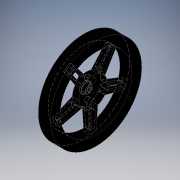
# Autodesk Inventor part: wheel
Saved by Autodesk Inventor 2016 (Build 200138000, 138)
## iProperties
Created: 2016-01-12
Part Number: wheel
Material: Generic
Document SubType Name: Modeling
Designer: jferner
Density: 1 g/cm^3
Appearance: Default
Author: jferner
Autodesk Inventor part; units mm, degrees
ref_plane "YZ Plane" through (0, 0, 0) normal (1, 0, 0) x (0, 1, 0)
sketch "Sketch1" plane through (0, 0, 0) normal (1, 0, 0) x (0, 1, 0)
  circle A0 centre (0, 0) radius 30
  circle A1 centre (0, 0) radius 23.65
  dimension "wheelDiameter" = 60
  dimension "wheelInnerDiameter" = 47.3
  constraints: 2 centre point, 2 coincident
  measures "wheelDiameter" diameter of A0
  measures "wheelInnerDiameter" diameter of A1
extrude "Extrusion1" add sketch "Sketch1" along normal mid plane 8
sketch "Sketch2" plane through (0, 0, 0) normal (1, 0, 0) x (0, 1, 0)
  circle A0 centre (0, 0) radius 9.4
  dimension "hubOuterDiameter" = 18.8
  constraints: 1 centre point, 1 coincident
  measures "hubOuterDiameter" diameter of A0
extrude "Extrusion2" add sketch "Sketch2" along normal mid plane 4.3
sketch "Sketch3" plane through (-2.15, 0, 0) normal (-1, 0, 0) x (0, 0, 1)
  circle A0 centre (0, 0) radius 1.22
  dimension "d7" = 2.44
  constraints: 1 centre point, 1 coincident
  measures "d7" diameter of A0
extrude "Extrusion3" cut sketch "Sketch3" against normal through all
sketch "Sketch4" plane through (-2.15, 0, 0) normal (-1, 0, 0) x (0, 0, 1)
  circle A0 centre (-6.3, 0) radius 1.6
  point P0 (0, 0)
  dimension "d10" = 3.2
  dimension "d11" = 6.3
  constraints: 1 centre point
  measures "d10" diameter of A0
  measures "d11" distance of point (0, 0) A0.centre
extrude "Extrusion4" cut sketch "Sketch4" against normal through all
pattern_circular "Circular Pattern1" count 2 over 360 about axis through (-2.15, 0, 0) along (1, 0, 0) of "Extrusion4"
sketch "Sketch5" plane through (-2.15, 0, 0) normal (-1, 0, 0) x (0, 0, 1)
  circle A0 centre (0, 0) radius 2.3
  circle A1 centre (0, 0) radius 1.22 projected
  circle A2 centre (0, 0) radius 3.5
  dimension "servoShaftDiameter" = 4.6
  dimension "d18" = 7
  constraints: 2 centre point, 2 coincident
  measures "servoShaftDiameter" diameter of A0
  measures "d18" diameter of A2
extrude "Extrusion5" add sketch "Sketch5" along normal blind 1.14 contours A2
sketch "Sketch7" plane through (-3.29, 0, 0) normal (-1, 0, 0) x (0, 0, 1)
  circle A0 centre (0, 0) radius 2.3
  dimension "d23" = 4.6
  constraints: 1 centre point, 1 coincident
  measures "d23" diameter of A0
extrude "Extrusion6" cut sketch "Sketch7" against normal blind 2.5
ref_plane "Work Plane2" through (0, 0, -9.4) normal (0, 0, 1) x (1, 0, 0)
sketch "Sketch9" plane through (0, 0, -9.4) normal (0, 0, 1) x (1, 0, 0)
  line L0 (2.15, 2.9) -> (-2.15, 2.9)
  line L1 (-2.15, 2.9) -> (-2.15, -2.9)
  line L2 (-2.15, -2.9) -> (2.15, -2.9)
  line L3 (2.15, -2.9) -> (2.15, 2.9)
  point P0 (0, 0)
  dimension "d24" = 2.15
  dimension "d25" = 4.3
  dimension "d26" = 5.8
  dimension "d27" = 2.9
  constraints: 8 end point, 2 parallel, 1 horizontal, 1 perpendicular
  measures "d24" distance from line of L1 point (0, 0)
  measures "d25" distance between parallel lines of L1 L3
  measures "d26" distance between parallel lines of L2 L0
  measures "d27" distance from line of L0 point (0, 0)
ref_plane "Work Plane3" through (0, 0, -23.65) normal (0, 0, 1) x (1, 0, 0)
sketch "Sketch10" plane through (0, 0, -23.65) normal (0, 0, 1) x (1, 0, 0)
  line L0 (-1.5, 2.5) -> (1.5, 2.5)
  line L1 (1.5, 2.5) -> (1.5, -2.5)
  line L2 (1.5, -2.5) -> (-1.5, -2.5)
  line L3 (-1.5, -2.5) -> (-1.5, 2.5)
  line L4 (0, 0) -> (2.563972, 0)
  line L5 (0, 0) -> (0, 2.208122)
  dimension "d28" = 3
  dimension "d29" = 5
  constraints: 12 end point, 2 horizontal, 2 parallel, 1 perpendicular, 1 vertical, 2 other
  measures "d28" distance between parallel lines of L1 L3
  measures "d29" distance of L0.end L1.end
sketch "Sketch10 outline for Loft1" plane through (0, 0, -23.65) normal (0, 0, 1) x (1, 0, 0)
  line L0 (-1.5, 2.5) -> (1.5, 2.5)
  line L1 (1.5, 2.5) -> (1.5, -2.5)
  line L2 (1.5, -2.5) -> (-1.5, -2.5)
  line L3 (-1.5, -2.5) -> (-1.5, 2.5)
sketch "Sketch9 outline for Loft1" plane through (0, 0, -9.4) normal (0, 0, 1) x (1, 0, 0)
  line L0 (2.15, -2.9) -> (2.15, 2.9)
  line L1 (-2.15, -2.9) -> (2.15, -2.9)
  line L2 (-2.15, 2.9) -> (-2.15, -2.9)
  line L3 (2.15, 2.9) -> (-2.15, 2.9)
loft "Loft1" add profiles "Sketch10 outline for Loft1", "Sketch9 outline for Loft1"
sketch "Sketch11" plane through (-2.15, 0, 0) normal (-1, 0, 0) x (0, 0, 1)
  line L0 (-23.517097, 2.503731) -> (-9.4, 2.9)
  line L1 (-9.4, 2.9) -> (-8.937253, 2.912989)
  circle A0 centre (0, 0) radius 9.4
  line L2 (-9.4, -2.9) -> (-9.4, 0)
  line L3 (-9.4, -2.9) -> (-8.941476, -2.9)
  line L4 (-9.4, -2.9) -> (-9.4, 2.9)
  constraints: 6 end point, 2 point on circle, 1 collinear, 1 perpendicular, 1 vertical
extrude "Extrusion7" add sketch "Sketch11" against normal up to surface contours L1 A0 L4 | A0 L3 L2 surface through (1.5, 2.5, -23.65) normal (-0.9989613, 0, 0.0455667)
sketch "Sketch12" plane through (0, 0, 0) normal (1, 0, 0) x (0, 1, 0)
  line L0 (1.509353, -11.641769) -> (1.240075, -21.234809)
  line L1 (-1.240075, -21.234809) -> (-1.509353, -11.641769)
  arc A0 (-1.240075, -21.234809) -> (1.240075, -21.234809) centre (0, -21.2) ccw
  arc A1 (1.509353, -11.641769) -> (-1.509353, -11.641769) centre (0, -11.9) ccw
  line L2 (0, 0) -> (0, -7.813594)
  line L3 (2.503731, -23.517097) -> (2.9, -9.4)
  line L4 (-2.503731, -23.517097) -> (-2.9, -9.4)
  dimension "d40" = 11.9
  dimension "d41" = 21.2
  dimension "d42" = 3.01871
  constraints: 6 end point, 4 point on circle, 2 centre point, 2 parallel, 2 point on line, 1 tangent, 1 vertical, 1 other
  measures "d40" distance of L2.start A1.centre
  measures "d41" distance of L2.start A0.centre
  measures "d42" distance of L1.end L0.start
extrude "Extrusion8" cut sketch "Sketch12" along normal through all both and the other way through all
pattern_circular "Circular Pattern3" count 5 over 360 about axis through (-2.15, 0, 0) along (1, 0, 0) of "Loft1", "Extrusion8", "Extrusion7"
equation "\"d23\" = servoShaftDiameter"
equation "\"d24\" = 0.5 * d25"
equation "\"d25\" = hubThickness"
equation "\"d27\" = 0.5 * d26"
equation "\"hubThickness\" = 4.3"
body "Solid1"
